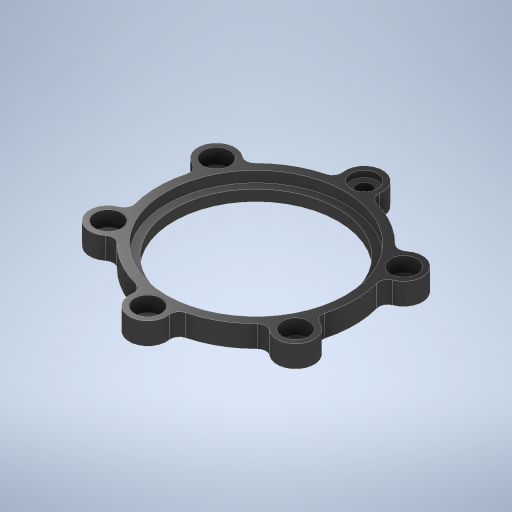
# Autodesk Inventor part: CrossRollerBearingOuterSupportStand
Saved by Autodesk Inventor 2024.2 (Build 282272000, 272)
## iProperties
Created: 2024-01-04
Part Number: CrossRollerBearingOuterSupportStand
Material: Aluminum 7075
Document SubType Name: Modeling
Designer: Masato Kubotera
Density: 2.81 g/cm^3
Appearance: Glossy - Black
Vendor: meviy
Mass: 7.60658 g
Surface Area: 35.3382 cm^2
Volume: 2.70697 cm^3
Author: Masato Kubotera
Autodesk Inventor part; units mm, degrees
ref_plane "YZ Plane" through (0, 0, 0) normal (1, 0, 0) x (0, 1, 0)
ref_plane "XZ Plane" through (0, 0, 0) normal (0, 1, 0) x (-1, 0, 0)
ref_plane "XY Plane" through (0, 0, 0) normal (0, 0, 1) x (1, 0, 0)
sketch "Sketch1" plane through (0, 0, 0) normal (0, 0, 1) x (1, 0, 0)
  circle A0 centre (0, 0) radius 20.5 construction
  line L0 (0, 0) -> (29, 0)
  circle A1 centre (24.75, 0) radius 4.25
  circle A2 centre (24.75, 0) radius 3 construction
  circle A3 centre (24.75, 0) radius 3.05 construction
  circle A4 centre (24.75, 0) radius 2.75 construction
  circle A5 centre (24.75, 0) radius 3.25 construction
  circle A6 centre (0, 0) radius 22.5
  circle A7 centre (12.375, 21.4341) radius 4.25
  circle A8 centre (-12.375, 21.4341) radius 4.25
  circle A9 centre (-24.75, 0) radius 4.25
  circle A10 centre (-12.375, -21.4341) radius 4.25
  circle A11 centre (12.375, -21.4341) radius 4.25
  point P0 (22.2374, -3.4277)
  point P1 (22.2374, 3.4277)
  point P2 (14.5, 25.1147)
  point P3 (-14.5, 25.1147)
  point P4 (-29, 0)
  point P5 (-14.5, -25.1147)
  point P6 (14.5, -25.1147)
  point P7 (14.0872, 17.5443)
  point P8 (8.1502, 20.972)
  point P9 (-8.1502, 20.972)
  point P10 (-14.0872, 17.5443)
  point P11 (-22.2374, -3.4277)
  point P12 (-22.2374, 3.4277)
  point P13 (-14.0872, -17.5443)
  point P14 (-8.1502, -20.972)
  point P15 (8.1502, -20.972)
  point P16 (14.0872, -17.5443)
  dimension "InsideDiameter" = 41
  dimension "SpacerOuterDiameter" = 6
  dimension "SpacerGap" = 0.05
  dimension "M3_HeadDiameter" = 5.5
  dimension "HeadDiameterThickness" = 0.5
  dimension "WallThickness" = 1
  dimension "d38" = 2
  dimension "d41" = 360
  constraints: 12 coincident, 6 centre point, 2 end point, 1 concentric, 1 horizontal, 1 point on line, 44 other
  measures "InsideDiameter" diameter of A0
  measures "SpacerOuterDiameter" diameter of A2
  measures "SpacerGap" radial gap between concentric circles of A3 A2
  measures "M3_HeadDiameter" diameter of A4
  measures "HeadDiameterThickness" radial gap between concentric circles of A5 A4
  measures "d38" radial gap between concentric circles of A6 A0
extrude "Extrusion1" add sketch "Sketch1" against normal blind 5
hole "Hole1" at (0, 0, 0) direction (0, 0, -1) diameter 37.5 end through all counterbore diameter 41 counterbore depth 2.5
hole "Hole2" at (24.75, 0, 0) at (12.375, -21.4341, 0) at (-12.375, -21.4341, 0) at (-12.375, 21.4341, 0) at (12.375, 21.4341, 0) direction (0, 0, -1) diameter 3.5 end through all counterbore diameter 6.1 counterbore depth 3.5
hole "Hole3" at (-24.75, 0, 0) direction (0, 0, -1) diameter 3.5 end through all counterbore diameter 6.1 counterbore depth 1.5
fillet "Fillet1" radius 2 12 edges at (22.2374, 3.4277, -2.5) (22.2374, -3.4277, -2.5) (14.0872, -17.5443, -2.5) (8.1502, -20.972, -2.5) (-14.0872, -17.5443, -2.5) (-8.1502, -20.972, -2.5) (-22.2374, -3.4277, -2.5) (-22.2374, 3.4277, -2.5) (-14.0872, 17.5443, -2.5) (-8.1502, 20.972, -2.5) (8.1502, 20.972, -2.5) (14.0872, 17.5443, -2.5)
equation "\"InsideDiameter_\" = InsideDiameter"
equation "\"SpacerDiameter\" = SpacerOuterDiameter + 2 * SpacerGap"
equation "\"d33\" = SpacerOuterDiameter + 2 * SpacerGap"
body "Solid1"
